Autodesk Inventor part; units mm, degrees
(part 2 of 2)
  spline S254 degree 2 poles (3.9442, -121.3977) (4.1617, -121.3977) (4.4669, -121.0893) (4.4669, -120.8718) knots 0 0 0 1 2 2 2
  line L190 (4.4669, -120.8718) -> (4.4669, -120.5244)
  spline S255 degree 2 poles (4.4669, -120.5244) (4.4669, -120.3036) (4.1617, -119.9984) (3.9442, -119.9984) knots 0 0 0 1 2 2 2
  line L191 (3.9442, -119.9984) -> (3.4214, -119.9984)
  spline S256 degree 2 poles (5.8662, -119.9984) (5.8662, -119.4692) (5.7623, -118.9464) knots 0 0 0 1 1 1
  spline S257 degree 2 poles (5.7623, -118.9464) (5.7039, -118.6542) (5.5286, -118.138) knots 0 0 0 1 1 1
  spline S258 degree 2 poles (5.5286, -118.138) (5.5156, -118.1088) (5.5156, -118.0763) knots 0 0 0 1 1 1
  spline S259 degree 2 poles (5.5156, -118.0763) (5.5156, -118.0049) (5.6227, -117.901) (5.6942, -117.901) knots 0 0 0 1 2 2 2
  spline S260 degree 2 poles (5.6942, -117.901) (5.8045, -117.901) (5.8435, -117.9821) knots 0 0 0 1 1 1
  spline S261 degree 2 poles (5.8435, -117.9821) (5.9896, -118.2971) (6.2169, -119.4205) (6.2169, -119.9984) knots 0 0 0 1 2 2 2
  spline S262 degree 2 poles (6.2169, -119.9984) (6.2169, -120.5795) (5.9896, -121.7029) (5.8435, -122.0179) knots 0 0 0 1 2 2 2
  spline S263 degree 2 poles (5.8435, -122.0179) (5.8045, -122.099) (5.6942, -122.099) knots 0 0 0 1 1 1
  spline S264 degree 2 poles (5.6942, -122.099) (5.626, -122.099) (5.5156, -121.9919) (5.5156, -121.9237) knots 0 0 0 1 2 2 2
  spline S265 degree 2 poles (5.5156, -121.9237) (5.5156, -121.8912) (5.5286, -121.862) knots 0 0 0 1 1 1
  spline S266 degree 2 poles (5.5286, -121.862) (5.7039, -121.3458) (5.7623, -121.0536) knots 0 0 0 1 1 1
  spline S267 degree 2 poles (5.7623, -121.0536) (5.8662, -120.5308) (5.8662, -119.9984) knots 0 0 0 1 1 1
  spline S268 degree 2 poles (34.4738, -116.6901) (34.4738, -116.5) (34.6529, -116.5) knots 0 0 0 1 1 1
  line L192 (34.6529, -116.5) -> (35.438, -116.5)
  spline S269 degree 2 poles (35.438, -116.5) (35.7355, -116.5) (36.1405, -116.949) (36.1405, -117.2713) knots 0 0 0 1 2 2 2
  line L193 (36.1405, -117.2713) -> (36.1405, -118.7287)
  spline S270 degree 2 poles (36.1405, -118.7287) (36.1405, -119.0482) (35.73, -119.5028) (35.438, -119.5028) knots 0 0 0 1 2 2 2
  line L194 (35.438, -119.5028) -> (34.6529, -119.5028)
  spline S271 degree 2 poles (34.6529, -119.5028) (34.4738, -119.5028) (34.4738, -119.3099) knots 0 0 0 1 1 1
  line L195 (34.4738, -119.3099) -> (34.4738, -116.6901)
  line L196 (34.8292, -116.8829) -> (34.8292, -119.1198)
  line L197 (34.8292, -119.1198) -> (35.438, -119.1198)
  spline S272 degree 2 poles (35.438, -119.1198) (35.5813, -119.1198) (35.7851, -118.8912) (35.7851, -118.7287) knots 0 0 0 1 2 2 2
  line L198 (35.7851, -118.7287) -> (35.7851, -117.2713)
  spline S273 degree 2 poles (35.7851, -117.2713) (35.7851, -117.1116) (35.5813, -116.8829) (35.438, -116.8829) knots 0 0 0 1 2 2 2
  line L199 (35.438, -116.8829) -> (34.8292, -116.8829)
  line L200 (36.6143, -119.3099) -> (36.6143, -116.6901)
  spline S274 degree 2 poles (36.6143, -116.6901) (36.6143, -116.5) (36.7934, -116.5) knots 0 0 0 1 1 1
  line L201 (36.7934, -116.5) -> (37.8402, -116.5)
  spline S275 degree 2 poles (37.8402, -116.5) (38.0165, -116.5) (38.0165, -116.6901) knots 0 0 0 1 1 1
  spline S276 degree 2 poles (38.0165, -116.6901) (38.0165, -116.8829) (37.8402, -116.8829) knots 0 0 0 1 1 1
  line L202 (37.8402, -116.8829) -> (36.9697, -116.8829)
  line L203 (36.9697, -116.8829) -> (36.9697, -117.6653)
  line L204 (36.9697, -117.6653) -> (37.5785, -117.6653)
  spline S277 degree 2 poles (37.5785, -117.6653) (37.7548, -117.6653) (37.7548, -117.8554) knots 0 0 0 1 1 1
  spline S278 degree 2 poles (37.7548, -117.8554) (37.7548, -118.0482) (37.5785, -118.0482) knots 0 0 0 1 1 1
  line L205 (37.5785, -118.0482) -> (36.9697, -118.0482)
  line L206 (36.9697, -118.0482) -> (36.9697, -119.1198)
  line L207 (36.9697, -119.1198) -> (37.8402, -119.1198)
  spline S279 degree 2 poles (37.8402, -119.1198) (38.0165, -119.1198) (38.0165, -119.3099) knots 0 0 0 1 1 1
  spline S280 degree 2 poles (38.0165, -119.3099) (38.0165, -119.5028) (37.8402, -119.5028) knots 0 0 0 1 1 1
  line L208 (37.8402, -119.5028) -> (36.7934, -119.5028)
  spline S281 degree 2 poles (36.7934, -119.5028) (36.6143, -119.5028) (36.6143, -119.3099) knots 0 0 0 1 1 1
  spline S282 degree 2 poles (38.4876, -116.6928) (38.4876, -116.5028) (38.6667, -116.5028) knots 0 0 0 1 1 1
  spline S283 degree 2 poles (38.6667, -116.5028) (38.843, -116.5028) (38.843, -116.6928) knots 0 0 0 1 1 1
  line L209 (38.843, -116.6928) -> (38.843, -119.1198)
  line L210 (38.843, -119.1198) -> (39.7135, -119.1198)
  spline S284 degree 2 poles (39.7135, -119.1198) (39.8898, -119.1198) (39.8898, -119.3099) knots 0 0 0 1 1 1
  spline S285 degree 2 poles (39.8898, -119.3099) (39.8898, -119.5028) (39.7135, -119.5028) knots 0 0 0 1 1 1
  line L211 (39.7135, -119.5028) -> (38.6667, -119.5028)
  spline S286 degree 2 poles (38.6667, -119.5028) (38.4876, -119.5028) (38.4876, -119.3099) knots 0 0 0 1 1 1
  line L212 (38.4876, -119.3099) -> (38.4876, -116.6928)
  spline S287 degree 2 poles (40.3609, -116.6901) (40.3609, -116.5) (40.5399, -116.5) knots 0 0 0 1 1 1
  line L213 (40.5399, -116.5) -> (41.8485, -116.5)
  spline S288 degree 2 poles (41.8485, -116.5) (42.0275, -116.5) (42.0275, -116.6901) knots 0 0 0 1 1 1
  spline S289 degree 2 poles (42.0275, -116.6901) (42.0275, -116.8829) (41.8485, -116.8829) knots 0 0 0 1 1 1
  line L214 (41.8485, -116.8829) -> (41.3719, -116.8829)
  line L215 (41.3719, -116.8829) -> (41.3719, -119.3099)
  spline S290 degree 2 poles (41.3719, -119.3099) (41.3719, -119.5028) (41.1956, -119.5028) knots 0 0 0 1 1 1
  spline S291 degree 2 poles (41.1956, -119.5028) (41.0165, -119.5028) (41.0165, -119.3099) knots 0 0 0 1 1 1
  line L216 (41.0165, -119.3099) -> (41.0165, -116.8829)
  line L217 (41.0165, -116.8829) -> (40.5399, -116.8829)
  spline S292 degree 2 poles (40.5399, -116.8829) (40.3609, -116.8829) (40.3609, -116.6901) knots 0 0 0 1 1 1
  spline S293 degree 2 poles (44.4298, -119.3099) (44.4298, -119.5028) (44.2507, -119.5028) knots 0 0 0 1 1 1
  spline S294 degree 2 poles (44.2507, -119.5028) (44.1212, -119.5028) (44.0799, -119.3705) knots 0 0 0 1 1 1
  line L218 (44.0799, -119.3705) -> (43.9008, -118.7755)
  line L219 (43.9008, -118.7755) -> (43.0275, -118.7755)
  line L220 (43.0275, -118.7755) -> (42.8485, -119.3705)
  spline S295 degree 2 poles (42.8485, -119.3705) (42.8099, -119.5028) (42.6804, -119.5028) knots 0 0 0 1 1 1
  spline S296 degree 2 poles (42.6804, -119.5028) (42.5014, -119.5028) (42.5014, -119.3099) knots 0 0 0 1 1 1
  spline S297 degree 2 poles (42.5014, -119.3099) (42.5014, -119.2769) (42.5096, -119.2521) knots 0 0 0 1 1 1
  line L221 (42.5096, -119.2521) -> (43.2893, -116.6515)
  spline S298 degree 2 poles (43.2893, -116.6515) (43.3333, -116.5028) (43.4656, -116.5028) knots 0 0 0 1 1 1
  spline S299 degree 2 poles (43.4656, -116.5028) (43.595, -116.5028) (43.6391, -116.646) knots 0 0 0 1 1 1
  line L222 (43.6391, -116.646) -> (44.4215, -119.2521)
  spline S300 degree 2 poles (44.4215, -119.2521) (44.4298, -119.2796) (44.4298, -119.3099) knots 0 0 0 1 1 1
  line L223 (43.4656, -117.1997) -> (43.1267, -118.3926)
  line L224 (43.1267, -118.3926) -> (43.8044, -118.3926)
  line L225 (43.8044, -118.3926) -> (43.4656, -117.1997)
  spline S301 degree 2 poles (48.1818, -118.7287) (48.1818, -119.0455) (47.7713, -119.5028) (47.4793, -119.5028) knots 0 0 0 1 2 2 2
  spline S302 degree 2 poles (47.4793, -119.5028) (46.978, -119.5028) (46.5895, -119.1722) knots 0 0 0 1 1 1
  spline S303 degree 2 poles (46.5895, -119.1722) (46.5152, -119.1116) (46.5152, -119.0179) knots 0 0 0 1 1 1
  spline S304 degree 2 poles (46.5152, -119.0179) (46.5152, -118.9435) (46.6171, -118.8278) (46.6942, -118.8278) knots 0 0 0 1 2 2 2
  spline S305 degree 2 poles (46.6942, -118.8278) (46.7383, -118.8278) (46.7989, -118.8664) knots 0 0 0 1 1 1
  spline S306 degree 2 poles (46.7989, -118.8664) (46.9063, -118.938) (47.157, -119.0647) knots 0 0 0 1 1 1
  spline S307 degree 2 poles (47.157, -119.0647) (47.2975, -119.1198) (47.4793, -119.1198) knots 0 0 0 1 1 1
  spline S308 degree 2 poles (47.4793, -119.1198) (47.6226, -119.1198) (47.8264, -118.8912) (47.8264, -118.7259) knots 0 0 0 1 2 2 2
  spline S309 degree 2 poles (47.8264, -118.7259) (47.8264, -118.489) (47.6309, -118.3788) knots 0 0 0 1 1 1
  line L226 (47.6309, -118.3788) -> (46.8953, -117.9601)
  spline S310 degree 2 poles (46.8953, -117.9601) (46.5152, -117.7424) (46.5152, -117.2713) knots 0 0 0 1 1 1
  spline S311 degree 2 poles (46.5152, -117.2713) (46.5152, -116.9573) (46.9256, -116.5) (47.2176, -116.5) knots 0 0 0 1 2 2 2
  spline S312 degree 2 poles (47.2176, -116.5) (47.697, -116.5) (47.9532, -116.668) knots 0 0 0 1 1 1
  spline S313 degree 2 poles (47.9532, -116.668) (48.0523, -116.7314) (48.0523, -116.8361) knots 0 0 0 1 1 1
  spline S314 degree 2 poles (48.0523, -116.8361) (48.0523, -116.9132) (47.9477, -117.0289) (47.8733, -117.0289) knots 0 0 0 1 2 2 2
  spline S315 degree 2 poles (47.8733, -117.0289) (47.843, -117.0289) (47.7989, -117.0096) knots 0 0 0 1 1 1
  spline S316 degree 2 poles (47.7989, -117.0096) (47.5041, -116.8829) (47.2176, -116.8829) knots 0 0 0 1 1 1
  spline S317 degree 2 poles (47.2176, -116.8829) (47.0744, -116.8829) (46.8705, -117.1088) (46.8705, -117.2713) knots 0 0 0 1 2 2 2
  spline S318 degree 2 poles (46.8705, -117.2713) (46.8705, -117.5165) (47.0606, -117.624) knots 0 0 0 1 1 1
  line L227 (47.0606, -117.624) -> (47.7989, -118.0427)
  spline S319 degree 2 poles (47.7989, -118.0427) (48.1818, -118.2603) (48.1818, -118.7287) knots 0 0 0 1 1 1
  spline S320 degree 2 poles (50.3223, -118.5826) (50.3223, -118.9628) (49.8347, -119.5028) (49.4904, -119.5028) knots 0 0 0 1 2 2 2
  spline S321 degree 2 poles (49.4904, -119.5028) (49.1433, -119.5028) (48.6556, -118.9628) (48.6556, -118.5826) knots 0 0 0 1 2 2 2
  line L228 (48.6556, -118.5826) -> (48.6556, -117.4174)
  spline S322 degree 2 poles (48.6556, -117.4174) (48.6556, -117.0399) (49.1405, -116.5) (49.4904, -116.5) knots 0 0 0 1 2 2 2
  spline S323 degree 2 poles (49.4904, -116.5) (49.8375, -116.5) (50.3223, -117.0372) (50.3223, -117.4174) knots 0 0 0 1 2 2 2
  line L229 (50.3223, -117.4174) -> (50.3223, -118.5826)
  line L230 (49.9669, -118.5826) -> (49.9669, -117.4174)
  spline S324 degree 2 poles (49.9669, -117.4174) (49.9669, -117.1915) (49.6887, -116.8829) (49.4904, -116.8829) knots 0 0 0 1 2 2 2
  spline S325 degree 2 poles (49.4904, -116.8829) (49.2893, -116.8829) (49.011, -117.1915) (49.011, -117.4174) knots 0 0 0 1 2 2 2
  line L231 (49.011, -117.4174) -> (49.011, -118.5826)
  spline S326 degree 2 poles (49.011, -118.5826) (49.011, -118.8113) (49.2893, -119.1198) (49.4904, -119.1198) knots 0 0 0 1 2 2 2
  spline S327 degree 2 poles (49.4904, -119.1198) (49.6887, -119.1198) (49.9669, -118.8113) (49.9669, -118.5826) knots 0 0 0 1 2 2 2
  spline S328 degree 2 poles (50.7961, -116.6928) (50.7961, -116.5028) (50.9752, -116.5028) knots 0 0 0 1 1 1
  spline S329 degree 2 poles (50.9752, -116.5028) (51.1515, -116.5028) (51.1515, -116.6928) knots 0 0 0 1 1 1
  line L232 (51.1515, -116.6928) -> (51.1515, -119.1198)
  line L233 (51.1515, -119.1198) -> (52.022, -119.1198)
  spline S330 degree 2 poles (52.022, -119.1198) (52.1983, -119.1198) (52.1983, -119.3099) knots 0 0 0 1 1 1
  spline S331 degree 2 poles (52.1983, -119.3099) (52.1983, -119.5028) (52.022, -119.5028) knots 0 0 0 1 1 1
  line L234 (52.022, -119.5028) -> (50.9752, -119.5028)
  spline S332 degree 2 poles (50.9752, -119.5028) (50.7961, -119.5028) (50.7961, -119.3099) knots 0 0 0 1 1 1
  line L235 (50.7961, -119.3099) -> (50.7961, -116.6928)
  spline S333 degree 2 poles (52.6694, -116.6928) (52.6694, -116.5028) (52.8485, -116.5028) knots 0 0 0 1 1 1
  spline S334 degree 2 poles (52.8485, -116.5028) (53.0248, -116.5028) (53.0248, -116.6928) knots 0 0 0 1 1 1
  line L236 (53.0248, -116.6928) -> (53.0248, -119.1198)
  line L237 (53.0248, -119.1198) -> (53.8953, -119.1198)
  spline S335 degree 2 poles (53.8953, -119.1198) (54.0716, -119.1198) (54.0716, -119.3099) knots 0 0 0 1 1 1
  spline S336 degree 2 poles (54.0716, -119.3099) (54.0716, -119.5028) (53.8953, -119.5028) knots 0 0 0 1 1 1
  line L238 (53.8953, -119.5028) -> (52.8485, -119.5028)
  spline S337 degree 2 poles (52.8485, -119.5028) (52.6694, -119.5028) (52.6694, -119.3099) knots 0 0 0 1 1 1
  line L239 (52.6694, -119.3099) -> (52.6694, -116.6928)
  line L240 (56.2094, -116.6928) -> (56.2094, -118.5826)
  spline S338 degree 2 poles (56.2094, -118.5826) (56.2094, -118.9628) (55.7218, -119.5028) (55.3774, -119.5028) knots 0 0 0 1 2 2 2
  spline S339 degree 2 poles (55.3774, -119.5028) (55.0303, -119.5028) (54.5427, -118.9628) (54.5427, -118.5826) knots 0 0 0 1 2 2 2
  line L241 (54.5427, -118.5826) -> (54.5427, -116.6928)
  spline S340 degree 2 poles (54.5427, -116.6928) (54.5427, -116.5028) (54.7218, -116.5028) knots 0 0 0 1 1 1
  spline S341 degree 2 poles (54.7218, -116.5028) (54.8981, -116.5028) (54.8981, -116.6928) knots 0 0 0 1 1 1
  line L242 (54.8981, -116.6928) -> (54.8981, -118.5826)
  spline S342 degree 2 poles (54.8981, -118.5826) (54.8981, -118.8113) (55.1763, -119.1198) (55.3774, -119.1198) knots 0 0 0 1 2 2 2
  spline S343 degree 2 poles (55.3774, -119.1198) (55.5758, -119.1198) (55.854, -118.8113) (55.854, -118.5826) knots 0 0 0 1 2 2 2
  line L243 (55.854, -118.5826) -> (55.854, -116.6928)
  spline S344 degree 2 poles (55.854, -116.6928) (55.854, -116.5028) (56.0331, -116.5028) knots 0 0 0 1 1 1
  spline S345 degree 2 poles (56.0331, -116.5028) (56.2094, -116.5028) (56.2094, -116.6928) knots 0 0 0 1 1 1
  spline S346 degree 2 poles (56.6832, -116.6901) (56.6832, -116.5) (56.8623, -116.5) knots 0 0 0 1 1 1
  line L244 (56.8623, -116.5) -> (58.1708, -116.5)
  spline S347 degree 2 poles (58.1708, -116.5) (58.3499, -116.5) (58.3499, -116.6901) knots 0 0 0 1 1 1
  spline S348 degree 2 poles (58.3499, -116.6901) (58.3499, -116.8829) (58.1708, -116.8829) knots 0 0 0 1 1 1
  line L245 (58.1708, -116.8829) -> (57.6942, -116.8829)
  line L246 (57.6942, -116.8829) -> (57.6942, -119.3099)
  spline S349 degree 2 poles (57.6942, -119.3099) (57.6942, -119.5028) (57.5179, -119.5028) knots 0 0 0 1 1 1
  spline S350 degree 2 poles (57.5179, -119.5028) (57.3388, -119.5028) (57.3388, -119.3099) knots 0 0 0 1 1 1
  line L247 (57.3388, -119.3099) -> (57.3388, -116.8829)
  line L248 (57.3388, -116.8829) -> (56.8623, -116.8829)
  spline S351 degree 2 poles (56.8623, -116.8829) (56.6832, -116.8829) (56.6832, -116.6901) knots 0 0 0 1 1 1
  spline S352 degree 2 poles (59.0028, -119.5028) (58.8237, -119.5028) (58.8237, -119.3099) knots 0 0 0 1 1 1
  line L249 (58.8237, -119.3099) -> (58.8237, -116.6928)
  spline S353 degree 2 poles (58.8237, -116.6928) (58.8237, -116.5028) (59.0028, -116.5028) knots 0 0 0 1 1 1
  spline S354 degree 2 poles (59.0028, -116.5028) (59.1791, -116.5028) (59.1791, -116.6928) knots 0 0 0 1 1 1
  line L250 (59.1791, -116.6928) -> (59.1791, -119.3099)
  spline S355 degree 2 poles (59.1791, -119.3099) (59.1791, -119.5028) (59.0028, -119.5028) knots 0 0 0 1 1 1
  spline S356 degree 2 poles (61.2948, -118.5826) (61.2948, -118.9628) (60.8072, -119.5028) (60.4628, -119.5028) knots 0 0 0 1 2 2 2
  spline S357 degree 2 poles (60.4628, -119.5028) (60.1157, -119.5028) (59.6281, -118.9628) (59.6281, -118.5826) knots 0 0 0 1 2 2 2
  line L251 (59.6281, -118.5826) -> (59.6281, -117.4174)
  spline S358 degree 2 poles (59.6281, -117.4174) (59.6281, -117.0399) (60.1129, -116.5) (60.4628, -116.5) knots 0 0 0 1 2 2 2
  spline S359 degree 2 poles (60.4628, -116.5) (60.8099, -116.5) (61.2948, -117.0372) (61.2948, -117.4174) knots 0 0 0 1 2 2 2
  line L252 (61.2948, -117.4174) -> (61.2948, -118.5826)
  line L253 (60.9394, -118.5826) -> (60.9394, -117.4174)
  spline S360 degree 2 poles (60.9394, -117.4174) (60.9394, -117.1915) (60.6612, -116.8829) (60.4628, -116.8829) knots 0 0 0 1 2 2 2
  spline S361 degree 2 poles (60.4628, -116.8829) (60.2617, -116.8829) (59.9835, -117.1915) (59.9835, -117.4174) knots 0 0 0 1 2 2 2
  line L254 (59.9835, -117.4174) -> (59.9835, -118.5826)
  spline S362 degree 2 poles (59.9835, -118.5826) (59.9835, -118.8113) (60.2617, -119.1198) (60.4628, -119.1198) knots 0 0 0 1 2 2 2
  spline S363 degree 2 poles (60.4628, -119.1198) (60.6612, -119.1198) (60.9394, -118.8113) (60.9394, -118.5826) knots 0 0 0 1 2 2 2
  line L255 (63.0799, -118.7011) -> (63.0799, -116.6928)
  spline S364 degree 2 poles (63.0799, -116.6928) (63.0799, -116.5028) (63.259, -116.5028) knots 0 0 0 1 1 1
  spline S365 degree 2 poles (63.259, -116.5028) (63.4353, -116.5028) (63.4353, -116.6928) knots 0 0 0 1 1 1
  line L256 (63.4353, -116.6928) -> (63.4353, -119.3099)
  spline S366 degree 2 poles (63.4353, -119.3099) (63.4353, -119.5028) (63.259, -119.5028) knots 0 0 0 1 1 1
  spline S367 degree 2 poles (63.259, -119.5028) (63.1488, -119.5028) (63.1019, -119.4036) knots 0 0 0 1 1 1
  line L257 (63.1019, -119.4036) -> (62.124, -117.2989)
  line L258 (62.124, -117.2989) -> (62.124, -119.3099)
  spline S368 degree 2 poles (62.124, -119.3099) (62.124, -119.5028) (61.9477, -119.5028) knots 0 0 0 1 1 1
  spline S369 degree 2 poles (61.9477, -119.5028) (61.7686, -119.5028) (61.7686, -119.3099) knots 0 0 0 1 1 1
  line L259 (61.7686, -119.3099) -> (61.7686, -116.6928)
  spline S370 degree 2 poles (61.7686, -116.6928) (61.7686, -116.5028) (61.9449, -116.5028) knots 0 0 0 1 1 1
  spline S371 degree 2 poles (61.9449, -116.5028) (62.0523, -116.5028) (62.1074, -116.6129) knots 0 0 0 1 1 1
  line L260 (62.1074, -116.6129) -> (63.0799, -118.7011)
  spline S372 degree 2 poles (65.5758, -118.7287) (65.5758, -119.0455) (65.1653, -119.5028) (64.8733, -119.5028) knots 0 0 0 1 2 2 2
  spline S373 degree 2 poles (64.8733, -119.5028) (64.3719, -119.5028) (63.9835, -119.1722) knots 0 0 0 1 1 1
  spline S374 degree 2 poles (63.9835, -119.1722) (63.9091, -119.1116) (63.9091, -119.0179) knots 0 0 0 1 1 1
  spline S375 degree 2 poles (63.9091, -119.0179) (63.9091, -118.9435) (64.011, -118.8278) (64.0882, -118.8278) knots 0 0 0 1 2 2 2
  spline S376 degree 2 poles (64.0882, -118.8278) (64.1322, -118.8278) (64.1928, -118.8664) knots 0 0 0 1 1 1
  spline S377 degree 2 poles (64.1928, -118.8664) (64.3003, -118.938) (64.551, -119.0647) knots 0 0 0 1 1 1
  spline S378 degree 2 poles (64.551, -119.0647) (64.6915, -119.1198) (64.8733, -119.1198) knots 0 0 0 1 1 1
  spline S379 degree 2 poles (64.8733, -119.1198) (65.0165, -119.1198) (65.2204, -118.8912) (65.2204, -118.7259) knots 0 0 0 1 2 2 2
  spline S380 degree 2 poles (65.2204, -118.7259) (65.2204, -118.489) (65.0248, -118.3788) knots 0 0 0 1 1 1
  line L261 (65.0248, -118.3788) -> (64.2893, -117.9601)
  spline S381 degree 2 poles (64.2893, -117.9601) (63.9091, -117.7424) (63.9091, -117.2713) knots 0 0 0 1 1 1
  spline S382 degree 2 poles (63.9091, -117.2713) (63.9091, -116.9573) (64.3196, -116.5) (64.6116, -116.5) knots 0 0 0 1 2 2 2
  spline S383 degree 2 poles (64.6116, -116.5) (65.0909, -116.5) (65.3471, -116.668) knots 0 0 0 1 1 1
  spline S384 degree 2 poles (65.3471, -116.668) (65.4463, -116.7314) (65.4463, -116.8361) knots 0 0 0 1 1 1
  spline S385 degree 2 poles (65.4463, -116.8361) (65.4463, -116.9132) (65.3416, -117.0289) (65.2672, -117.0289) knots 0 0 0 1 2 2 2
  spline S386 degree 2 poles (65.2672, -117.0289) (65.2369, -117.0289) (65.1928, -117.0096) knots 0 0 0 1 1 1
  spline S387 degree 2 poles (65.1928, -117.0096) (64.8981, -116.8829) (64.6116, -116.8829) knots 0 0 0 1 1 1
  spline S388 degree 2 poles (64.6116, -116.8829) (64.4683, -116.8829) (64.2645, -117.1088) (64.2645, -117.2713) knots 0 0 0 1 2 2 2
  spline S389 degree 2 poles (64.2645, -117.2713) (64.2645, -117.5165) (64.4545, -117.624) knots 0 0 0 1 1 1
  line L262 (64.4545, -117.624) -> (65.1928, -118.0427)
  spline S390 degree 2 poles (65.1928, -118.0427) (65.5758, -118.2603) (65.5758, -118.7287) knots 0 0 0 1 1 1
  spline S391 degree 2 poles (40.1878, -123.1609) (40.0994, -123.1609) (40.0705, -123.0774) knots 0 0 0 1 1 1
  line L263 (40.0705, -123.0774) -> (39.5129, -121.5588)
  spline S392 degree 2 poles (39.5129, -121.5588) (39.5064, -121.5427) (39.5064, -121.5218) knots 0 0 0 1 1 1
  spline S393 degree 2 poles (39.5064, -121.5218) (39.5064, -121.4109) (39.627, -121.4109) knots 0 0 0 1 1 1
  spline S394 degree 2 poles (39.627, -121.4109) (39.7153, -121.4109) (39.7427, -121.4848) knots 0 0 0 1 1 1
  line L264 (39.7427, -121.4848) -> (40.1878, -122.7511)
  line L265 (40.1878, -122.7511) -> (40.6329, -121.4848)
  spline S395 degree 2 poles (40.6329, -121.4848) (40.6602, -121.4109) (40.7486, -121.4109) knots 0 0 0 1 1 1
  spline S396 degree 2 poles (40.7486, -121.4109) (40.8691, -121.4109) (40.8691, -121.5218) knots 0 0 0 1 1 1
  spline S397 degree 2 poles (40.8691, -121.5218) (40.8691, -121.5427) (40.8627, -121.5588) knots 0 0 0 1 1 1
  line L266 (40.8627, -121.5588) -> (40.3051, -123.0774)
  spline S398 degree 2 poles (40.3051, -123.0774) (40.2746, -123.1609) (40.1878, -123.1609) knots 0 0 0 1 1 1
  spline S399 degree 2 poles (41.3432, -123.1609) (41.2227, -123.1609) (41.2227, -123.0484) knots 0 0 0 1 1 1
  line L267 (41.2227, -123.0484) -> (41.2227, -121.5218)
  spline S400 degree 2 poles (41.2227, -121.5218) (41.2227, -121.4109) (41.3432, -121.4109) knots 0 0 0 1 1 1
  spline S401 degree 2 poles (41.3432, -121.4109) (41.4637, -121.4109) (41.4637, -121.5218) knots 0 0 0 1 1 1
  line L268 (41.4637, -121.5218) -> (41.4637, -123.0484)
  spline S402 degree 2 poles (41.4637, -123.0484) (41.4637, -123.1609) (41.3432, -123.1609) knots 0 0 0 1 1 1
  spline S403 degree 2 poles (42.4777, -123.1609) (42.3893, -123.1609) (42.3604, -123.0774) knots 0 0 0 1 1 1
  line L269 (42.3604, -123.0774) -> (41.8028, -121.5588)
  spline S404 degree 2 poles (41.8028, -121.5588) (41.7964, -121.5427) (41.7964, -121.5218) knots 0 0 0 1 1 1
  spline S405 degree 2 poles (41.7964, -121.5218) (41.7964, -121.4109) (41.9169, -121.4109) knots 0 0 0 1 1 1
  spline S406 degree 2 poles (41.9169, -121.4109) (42.0053, -121.4109) (42.0326, -121.4848) knots 0 0 0 1 1 1
  line L270 (42.0326, -121.4848) -> (42.4777, -122.7511)
  line L271 (42.4777, -122.7511) -> (42.9229, -121.4848)
  spline S407 degree 2 poles (42.9229, -121.4848) (42.9502, -121.4109) (43.0386, -121.4109) knots 0 0 0 1 1 1
  spline S408 degree 2 poles (43.0386, -121.4109) (43.1591, -121.4109) (43.1591, -121.5218) knots 0 0 0 1 1 1
  spline S409 degree 2 poles (43.1591, -121.5218) (43.1591, -121.5427) (43.1527, -121.5588) knots 0 0 0 1 1 1
  line L272 (43.1527, -121.5588) -> (42.595, -123.0774)
  spline S410 degree 2 poles (42.595, -123.0774) (42.5645, -123.1609) (42.4777, -123.1609) knots 0 0 0 1 1 1
  spline S411 degree 2 poles (44.8753, -123.0484) (44.8753, -123.1609) (44.7548, -123.1609) knots 0 0 0 1 1 1
  spline S412 degree 2 poles (44.7548, -123.1609) (44.6664, -123.1609) (44.6391, -123.0854) knots 0 0 0 1 1 1
  line L273 (44.6391, -123.0854) -> (44.5106, -122.7367)
  line L274 (44.5106, -122.7367) -> (43.8758, -122.7367)
  line L275 (43.8758, -122.7367) -> (43.7489, -123.0854)
  spline S413 degree 2 poles (43.7489, -123.0854) (43.7215, -123.1609) (43.6331, -123.1609) knots 0 0 0 1 1 1
  spline S414 degree 2 poles (43.6331, -123.1609) (43.5126, -123.1609) (43.5126, -123.0484) knots 0 0 0 1 1 1
  spline S415 degree 2 poles (43.5126, -123.0484) (43.5126, -123.0275) (43.5191, -123.0131) knots 0 0 0 1 1 1
  line L276 (43.5191, -123.0131) -> (44.0735, -121.5315)
  spline S416 degree 2 poles (44.0735, -121.5315) (44.1072, -121.4109) (44.194, -121.4109) knots 0 0 0 1 1 1
  spline S417 degree 2 poles (44.194, -121.4109) (44.2808, -121.4109) (44.3113, -121.4929) knots 0 0 0 1 1 1
  line L277 (44.3113, -121.4929) -> (44.8689, -123.0131)
  spline S418 degree 2 poles (44.8689, -123.0131) (44.8753, -123.0292) (44.8753, -123.0484) knots 0 0 0 1 1 1
  line L278 (44.194, -121.8175) -> (43.9465, -122.5133)
  line L279 (43.9465, -122.5133) -> (44.4415, -122.5133)
  line L280 (44.4415, -122.5133) -> (44.194, -121.8175)
  spline S419 degree 2 poles (47.7358, -123.0484) (47.7358, -123.1609) (47.6152, -123.1609) knots 0 0 0 1 1 1
  spline S420 degree 2 poles (47.6152, -123.1609) (47.5269, -123.1609) (47.4995, -123.0854) knots 0 0 0 1 1 1
  line L281 (47.4995, -123.0854) -> (47.371, -122.7367)
  line L282 (47.371, -122.7367) -> (46.7362, -122.7367)
  line L283 (46.7362, -122.7367) -> (46.6093, -123.0854)
  spline S421 degree 2 poles (46.6093, -123.0854) (46.582, -123.1609) (46.4936, -123.1609) knots 0 0 0 1 1 1
  spline S422 degree 2 poles (46.4936, -123.1609) (46.373, -123.1609) (46.373, -123.0484) knots 0 0 0 1 1 1
  spline S423 degree 2 poles (46.373, -123.0484) (46.373, -123.0275) (46.3795, -123.0131) knots 0 0 0 1 1 1
  line L284 (46.3795, -123.0131) -> (46.9339, -121.5315)
  spline S424 degree 2 poles (46.9339, -121.5315) (46.9676, -121.4109) (47.0544, -121.4109) knots 0 0 0 1 1 1
  spline S425 degree 2 poles (47.0544, -121.4109) (47.1412, -121.4109) (47.1717, -121.4929) knots 0 0 0 1 1 1
  line L285 (47.1717, -121.4929) -> (47.7293, -123.0131)
  spline S426 degree 2 poles (47.7293, -123.0131) (47.7358, -123.0292) (47.7358, -123.0484) knots 0 0 0 1 1 1
  line L286 (47.0544, -121.8175) -> (46.8069, -122.5133)
  line L287 (46.8069, -122.5133) -> (47.3019, -122.5133)
  line L288 (47.3019, -122.5133) -> (47.0544, -121.8175)
  spline S427 degree 2 poles (46.7475, -120.8405) (46.7475, -120.7312) (46.868, -120.7312) knots 0 0 0 1 1 1
  spline S428 degree 2 poles (46.868, -120.7312) (46.9082, -120.7312) (46.9307, -120.7456) knots 0 0 0 1 1 1
  line L289 (46.9307, -120.7456) -> (47.3067, -121.0028)
  spline S429 degree 2 poles (47.3067, -121.0028) (47.3613, -121.0397) (47.3613, -121.096) knots 0 0 0 1 1 1
  spline S430 degree 2 poles (47.3613, -121.096) (47.3613, -121.2084) (47.2408, -121.2084) knots 0 0 0 1 1 1
  spline S431 degree 2 poles (47.2408, -121.2084) (47.199, -121.2084) (47.1685, -121.186) knots 0 0 0 1 1 1
  line L290 (47.1685, -121.186) -> (46.8021, -120.9369)
  spline S432 degree 2 poles (46.8021, -120.9369) (46.7475, -120.8999) (46.7475, -120.8405) knots 0 0 0 1 1 1
  spline S433 degree 2 poles (49.354, -123.1609) (49.2335, -123.1609) (49.2335, -123.0484) knots 0 0 0 1 1 1
  line L291 (49.2335, -123.0484) -> (49.2335, -121.5218)
  spline S434 degree 2 poles (49.2335, -121.5218) (49.2335, -121.4109) (49.354, -121.4109) knots 0 0 0 1 1 1
  spline S435 degree 2 poles (49.354, -121.4109) (49.4745, -121.4109) (49.4745, -121.5218) knots 0 0 0 1 1 1
  line L292 (49.4745, -121.5218) -> (49.4745, -123.0484)
  spline S436 degree 2 poles (49.4745, -123.0484) (49.4745, -123.1609) (49.354, -123.1609) knots 0 0 0 1 1 1
  line L293 (50.7424, -122.6933) -> (50.7424, -121.5218)
  spline S437 degree 2 poles (50.7424, -121.5218) (50.7424, -121.4109) (50.8629, -121.4109) knots 0 0 0 1 1 1
  spline S438 degree 2 poles (50.8629, -121.4109) (50.9835, -121.4109) (50.9835, -121.5218) knots 0 0 0 1 1 1
  line L294 (50.9835, -121.5218) -> (50.9835, -123.0484)
  spline S439 degree 2 poles (50.9835, -123.0484) (50.9835, -123.1609) (50.8629, -123.1609) knots 0 0 0 1 1 1
  spline S440 degree 2 poles (50.8629, -123.1609) (50.7906, -123.1609) (50.7697, -123.1191) knots 0 0 0 1 1 1
  line L295 (50.7697, -123.1191) -> (50.0482, -121.8753)
  line L296 (50.0482, -121.8753) -> (50.0482, -123.0484)
  spline S441 degree 2 poles (50.0482, -123.0484) (50.0482, -123.1609) (49.9277, -123.1609) knots 0 0 0 1 1 1
  spline S442 degree 2 poles (49.9277, -123.1609) (49.8072, -123.1609) (49.8072, -123.0484) knots 0 0 0 1 1 1
  line L297 (49.8072, -123.0484) -> (49.8072, -121.5218)
  spline S443 degree 2 poles (49.8072, -121.5218) (49.8072, -121.4109) (49.9277, -121.4109) knots 0 0 0 1 1 1
  spline S444 degree 2 poles (49.9277, -121.4109) (49.9984, -121.4109) (50.037, -121.4736) knots 0 0 0 1 1 1
  line L298 (50.037, -121.4736) -> (50.7424, -122.6933)
  spline S445 degree 2 poles (52.5085, -122.6242) (52.5085, -122.8476) (52.163, -123.1609) (51.9203, -123.1609) knots 0 0 0 1 2 2 2
  spline S446 degree 2 poles (51.9203, -123.1609) (51.6761, -123.1609) (51.3322, -122.8476) (51.3322, -122.6242) knots 0 0 0 1 2 2 2
  line L299 (51.3322, -122.6242) -> (51.3322, -121.9444)
  spline S447 degree 2 poles (51.3322, -121.9444) (51.3322, -121.7227) (51.6761, -121.4093) (51.9203, -121.4093) knots 0 0 0 1 2 2 2
  spline S448 degree 2 poles (51.9203, -121.4093) (52.1646, -121.4093) (52.5085, -121.7211) (52.5085, -121.9444) knots 0 0 0 1 2 2 2
  line L300 (52.5085, -121.9444) -> (52.5085, -122.6242)
  line L301 (52.2674, -122.6242) -> (52.2674, -121.9444)
  spline S449 degree 2 poles (52.2674, -121.9444) (52.2674, -121.8143) (52.0666, -121.6327) (51.9203, -121.6327) knots 0 0 0 1 2 2 2
  spline S450 degree 2 poles (51.9203, -121.6327) (51.7741, -121.6327) (51.5732, -121.8143) (51.5732, -121.9444) knots 0 0 0 1 2 2 2
  line L302 (51.5732, -121.9444) -> (51.5732, -122.6242)
  spline S451 degree 2 poles (51.5732, -122.6242) (51.5732, -122.756) (51.7741, -122.9376) (51.9203, -122.9376) knots 0 0 0 1 2 2 2
  spline S452 degree 2 poles (51.9203, -122.9376) (52.0666, -122.9376) (52.2674, -122.756) (52.2674, -122.6242) knots 0 0 0 1 2 2 2
  spline S453 degree 2 poles (53.5386, -123.1609) (53.4502, -123.1609) (53.4213, -123.0774) knots 0 0 0 1 1 1
  line L303 (53.4213, -123.0774) -> (52.8636, -121.5588)
  spline S454 degree 2 poles (52.8636, -121.5588) (52.8572, -121.5427) (52.8572, -121.5218) knots 0 0 0 1 1 1
  spline S455 degree 2 poles (52.8572, -121.5218) (52.8572, -121.4109) (52.9777, -121.4109) knots 0 0 0 1 1 1
  spline S456 degree 2 poles (52.9777, -121.4109) (53.0661, -121.4109) (53.0934, -121.4848) knots 0 0 0 1 1 1
  line L304 (53.0934, -121.4848) -> (53.5386, -122.7511)
  line L305 (53.5386, -122.7511) -> (53.9837, -121.4848)
  spline S457 degree 2 poles (53.9837, -121.4848) (54.011, -121.4109) (54.0994, -121.4109) knots 0 0 0 1 1 1
  spline S458 degree 2 poles (54.0994, -121.4109) (54.2199, -121.4109) (54.2199, -121.5218) knots 0 0 0 1 1 1
  spline S459 degree 2 poles (54.2199, -121.5218) (54.2199, -121.5427) (54.2135, -121.5588) knots 0 0 0 1 1 1
  line L306 (54.2135, -121.5588) -> (53.6559, -123.0774)
  spline S460 degree 2 poles (53.6559, -123.0774) (53.6253, -123.1609) (53.5386, -123.1609) knots 0 0 0 1 1 1
  spline S461 degree 2 poles (55.9362, -123.0484) (55.9362, -123.1609) (55.8157, -123.1609) knots 0 0 0 1 1 1
  spline S462 degree 2 poles (55.8157, -123.1609) (55.7273, -123.1609) (55.7, -123.0854) knots 0 0 0 1 1 1
  line L307 (55.7, -123.0854) -> (55.5714, -122.7367)
  line L308 (55.5714, -122.7367) -> (54.9366, -122.7367)
  line L309 (54.9366, -122.7367) -> (54.8097, -123.0854)
  spline S463 degree 2 poles (54.8097, -123.0854) (54.7824, -123.1609) (54.694, -123.1609) knots 0 0 0 1 1 1
  spline S464 degree 2 poles (54.694, -123.1609) (54.5735, -123.1609) (54.5735, -123.0484) knots 0 0 0 1 1 1
  spline S465 degree 2 poles (54.5735, -123.0484) (54.5735, -123.0275) (54.5799, -123.0131) knots 0 0 0 1 1 1
  line L310 (54.5799, -123.0131) -> (55.1343, -121.5315)
  spline S466 degree 2 poles (55.1343, -121.5315) (55.168, -121.4109) (55.2548, -121.4109) knots 0 0 0 1 1 1
  spline S467 degree 2 poles (55.2548, -121.4109) (55.3416, -121.4109) (55.3721, -121.4929) knots 0 0 0 1 1 1
  line L311 (55.3721, -121.4929) -> (55.9298, -123.0131)
  spline S468 degree 2 poles (55.9298, -123.0131) (55.9362, -123.0292) (55.9362, -123.0484) knots 0 0 0 1 1 1
  line L312 (55.2548, -121.8175) -> (55.0073, -122.5133)
  line L313 (55.0073, -122.5133) -> (55.5023, -122.5133)
  line L314 (55.5023, -122.5133) -> (55.2548, -121.8175)
  spline S469 degree 2 poles (56.6899, -123.5) (56.5693, -123.5) (56.5693, -123.3875) knots 0 0 0 1 1 1
  spline S470 degree 2 poles (56.5693, -123.3875) (56.5693, -123.3747) (56.64, -123.14) knots 0 0 0 1 1 1
  spline S471 degree 2 poles (56.64, -123.14) (56.4986, -123.1095) (56.2897, -122.8636) (56.2897, -122.7078) knots 0 0 0 1 2 2 2
  line L315 (56.2897, -122.7078) -> (56.2897, -121.8593)
  spline S472 degree 2 poles (56.2897, -121.8593) (56.2897, -121.6729) (56.579, -121.4093) (56.7831, -121.4093) knots 0 0 0 1 2 2 2
  line L316 (56.7831, -121.4093) -> (57.1575, -121.4093)
  spline S473 degree 2 poles (57.1575, -121.4093) (57.278, -121.4093) (57.278, -121.5202) knots 0 0 0 1 1 1
  spline S474 degree 2 poles (57.278, -121.5202) (57.278, -121.6327) (57.1575, -121.6327) knots 0 0 0 1 1 1
  line L317 (57.1575, -121.6327) -> (56.7831, -121.6327)
  spline S475 degree 2 poles (56.7831, -121.6327) (56.6368, -121.6327) (56.5645, -121.7468) knots 0 0 0 1 1 1
  spline S476 degree 2 poles (56.5645, -121.7468) (56.5308, -121.7982) (56.5308, -121.8593) knots 0 0 0 1 1 1
  line L318 (56.5308, -121.8593) -> (56.5308, -122.7094)
  spline S477 degree 2 poles (56.5308, -122.7094) (56.5308, -122.8026) (56.6786, -122.9376) (56.7831, -122.9376) knots 0 0 0 1 2 2 2
  line L319 (56.7831, -122.9376) -> (57.1575, -122.9376)
  spline S478 degree 2 poles (57.1575, -122.9376) (57.278, -122.9376) (57.278, -123.0484) knots 0 0 0 1 1 1
  spline S479 degree 2 poles (57.278, -123.0484) (57.278, -123.1609) (57.1575, -123.1609) knots 0 0 0 1 1 1
  line L320 (57.1575, -123.1609) -> (56.8779, -123.1609)
  line L321 (56.8779, -123.1609) -> (56.8072, -123.4164)
  spline S480 degree 2 poles (56.8072, -123.4164) (56.7831, -123.5) (56.6899, -123.5) knots 0 0 0 1 1 1
  spline S481 degree 2 poles (58.9878, -123.0484) (58.9878, -123.1609) (58.8673, -123.1609) knots 0 0 0 1 1 1
  spline S482 degree 2 poles (58.8673, -123.1609) (58.7789, -123.1609) (58.7516, -123.0854) knots 0 0 0 1 1 1
  line L322 (58.7516, -123.0854) -> (58.623, -122.7367)
  line L323 (58.623, -122.7367) -> (57.9883, -122.7367)
  line L324 (57.9883, -122.7367) -> (57.8613, -123.0854)
  spline S483 degree 2 poles (57.8613, -123.0854) (57.834, -123.1609) (57.7456, -123.1609) knots 0 0 0 1 1 1
  spline S484 degree 2 poles (57.7456, -123.1609) (57.6251, -123.1609) (57.6251, -123.0484) knots 0 0 0 1 1 1
  spline S485 degree 2 poles (57.6251, -123.0484) (57.6251, -123.0275) (57.6315, -123.0131) knots 0 0 0 1 1 1
  line L325 (57.6315, -123.0131) -> (58.186, -121.5315)
  spline S486 degree 2 poles (58.186, -121.5315) (58.2197, -121.4109) (58.3065, -121.4109) knots 0 0 0 1 1 1
  spline S487 degree 2 poles (58.3065, -121.4109) (58.3933, -121.4109) (58.4238, -121.4929) knots 0 0 0 1 1 1
  line L326 (58.4238, -121.4929) -> (58.9814, -123.0131)
  spline S488 degree 2 poles (58.9814, -123.0131) (58.9878, -123.0292) (58.9878, -123.0484) knots 0 0 0 1 1 1
  spline S489 degree 2 poles (58.4929, -121.1233) (58.4254, -121.1233) (58.3579, -121.0895) knots 0 0 0 1 1 1
  spline S490 degree 2 poles (58.3579, -121.0895) (58.2888, -121.0494) (58.2518, -121.0285) knots 0 0 0 1 1 1
  spline S491 degree 2 poles (58.2518, -121.0285) (58.2229, -121.0172) (58.1699, -120.9787) knots 0 0 0 1 1 1
  spline S492 degree 2 poles (58.1699, -120.9787) (58.1361, -120.9545) (58.1201, -120.9545) knots 0 0 0 1 1 1
  spline S493 degree 2 poles (58.1201, -120.9545) (58.0911, -120.9545) (57.9803, -121.0381) (57.9337, -121.0381) knots 0 0 0 1 2 2 2
  spline S494 degree 2 poles (57.9337, -121.0381) (57.8854, -121.0381) (57.8115, -120.9722) (57.8115, -120.9272) knots 0 0 0 1 2 2 2
  spline S495 degree 2 poles (57.8115, -120.9272) (57.8115, -120.871) (57.9047, -120.8308) knots 0 0 0 1 1 1
  spline S496 degree 2 poles (57.9047, -120.8308) (57.9529, -120.7762) (57.9899, -120.7585) knots 0 0 0 1 1 1
  spline S497 degree 2 poles (57.9899, -120.7585) (58.0429, -120.7312) (58.1201, -120.7312) knots 0 0 0 1 1 1
  spline S498 degree 2 poles (58.1201, -120.7312) (58.1811, -120.7312) (58.2518, -120.7649) knots 0 0 0 1 1 1
  spline S499 degree 2 poles (58.2518, -120.7649) (58.3017, -120.7922) (58.3499, -120.8196) knots 0 0 0 1 1 1
  spline S500 degree 2 poles (58.3499, -120.8196) (58.382, -120.8324) (58.4399, -120.8742) knots 0 0 0 1 1 1
  spline S501 degree 2 poles (58.4399, -120.8742) (58.4768, -120.9015) (58.4929, -120.9015) knots 0 0 0 1 1 1
  spline S502 degree 2 poles (58.4929, -120.9015) (58.5218, -120.9015) (58.6343, -120.8163) (58.6793, -120.8163) knots 0 0 0 1 2 2 2
  spline S503 degree 2 poles (58.6793, -120.8163) (58.7998, -120.8163) (58.7998, -120.9272) knots 0 0 0 1 1 1
  spline S504 degree 2 poles (58.7998, -120.9272) (58.7998, -120.9787) (58.75, -121.0188) knots 0 0 0 1 1 1
  spline S505 degree 2 poles (58.75, -121.0188) (58.713, -121.0429) (58.6761, -121.0686) knots 0 0 0 1 1 1
  spline S506 degree 2 poles (58.6761, -121.0686) (58.5941, -121.1233) (58.4929, -121.1233) knots 0 0 0 1 1 1
  line L327 (58.3065, -121.8175) -> (58.059, -122.5133)
  line L328 (58.059, -122.5133) -> (58.5539, -122.5133)
  line L329 (58.5539, -122.5133) -> (58.3065, -121.8175)
  spline S507 degree 2 poles (60.5177, -122.6242) (60.5177, -122.8476) (60.1722, -123.1609) (59.9295, -123.1609) knots 0 0 0 1 2 2 2
  spline S508 degree 2 poles (59.9295, -123.1609) (59.6853, -123.1609) (59.3414, -122.8476) (59.3414, -122.6242) knots 0 0 0 1 2 2 2
  line L330 (59.3414, -122.6242) -> (59.3414, -121.9444)
  spline S509 degree 2 poles (59.3414, -121.9444) (59.3414, -121.7227) (59.6853, -121.4093) (59.9295, -121.4093) knots 0 0 0 1 2 2 2
  spline S510 degree 2 poles (59.9295, -121.4093) (60.1738, -121.4093) (60.5177, -121.7211) (60.5177, -121.9444) knots 0 0 0 1 2 2 2
  line L331 (60.5177, -121.9444) -> (60.5177, -122.6242)
  line L332 (60.2766, -122.6242) -> (60.2766, -121.9444)
  spline S511 degree 2 poles (60.2766, -121.9444) (60.2766, -121.8143) (60.0758, -121.6327) (59.9295, -121.6327) knots 0 0 0 1 2 2 2
  spline S512 degree 2 poles (59.9295, -121.6327) (59.7833, -121.6327) (59.5824, -121.8143) (59.5824, -121.9444) knots 0 0 0 1 2 2 2
  line L333 (59.5824, -121.9444) -> (59.5824, -122.6242)
  spline S513 degree 2 poles (59.5824, -122.6242) (59.5824, -122.756) (59.7833, -122.9376) (59.9295, -122.9376) knots 0 0 0 1 2 2 2
  spline S514 degree 2 poles (59.9295, -122.9376) (60.0758, -122.9376) (60.2766, -122.756) (60.2766, -122.6242) knots 0 0 0 1 2 2 2
  point P0 (0, 0)
  point P1 (-70.4, -120)
  point P2 (30, -120)
  point P3 (27, -116.5)
  point P4 (66.5, -121.5)
  point P5 (70, -120)
  dimension "d58" = 33
  dimension "d59" = 40
  dimension "d60" = 4
  dimension "d61" = 7
  dimension "d62" = 3
  dimension "d63" = 10
  dimension "d64" = 1.5
  dimension "d65" = 9.6
  constraints: 5 midpoint, 2 end point, 2 horizontal, 1 horizontal alignment, 1 parallel, 1 perpendicular, 1 point on line, 7 other
  measures "d58" distance from line of point (66.5, -121.5) L0
  measures "d59" distance from line of point (70, -120) L1
  measures "d60" distance between parallel lines of L6 L3
  measures "d61" distance between parallel lines of L6 L5
  measures "d62" distance from line of L1 point (27, -116.5)
  measures "d63" distance between parallel lines of L9 L7
  measures "d64" distance between parallel lines of L10 L4
  measures "d65" distance from line of L11 point (-70.4, -120)
emboss "Relevo1" sketch "Esboço3" operation cut depth 0.1 direction (0, 0, -1)
